Autodesk Fusion 360 part; units mm, degrees
(part 2 of 2)
sketch "side_face" plane through (8.1771, 0, 4.1664) normal (0.891007, 0, 0.45399) x (0, 1, 0) in component "sides"
  line L0 (-20, -43.5513) -> (-23, -43.5513)
  line L1 (-23, -43.5513) -> (-23, -35.5513)
  line L2 (-23, -35.5513) -> (-20, -35.5513)
  line L3 (-20, -35.5513) -> (-20, -43.5513)
  line L4 (20, -35.5513) -> (23, -35.5513)
  line L5 (23, -35.5513) -> (23, -43.5513)
  line L6 (23, -43.5513) -> (20, -43.5513)
  line L7 (20, -43.5513) -> (20, -35.5513)
  line L8 (22.4714, -88.3181) -> (61.9525, -140.4776)
  line L9 (61.9525, -140.4776) -> (67.9525, -140.4776)
  line L10 (67.9525, -140.4776) -> (67.9525, -143.8445)
  line L11 (67.9525, -143.8445) -> (73.9525, -143.8445)
  line L12 (73.9525, -143.8445) -> (73.9525, -140.4776)
  line L13 (73.9525, -140.4776) -> (23, -28.2449)
  line L14 (23, -28.2449) -> (-23, -28.2449)
  line L15 (-23, -28.2449) -> (-73.9525, -140.4776)
  line L16 (-73.9525, -140.4776) -> (-73.9525, -143.8445)
  line L17 (-73.9525, -143.8445) -> (-67.9525, -143.8445)
  line L18 (-67.9525, -143.8445) -> (-67.9525, -140.4776)
  line L19 (-67.9525, -140.4776) -> (-61.9525, -140.4776)
  line L20 (-61.9525, -140.4776) -> (-22.4714, -88.3181)
  ellipse E0 centre (-14.8502, -95.5845) end of major axis (-14.8502, -84.3612) minor radius 10 (-14.8502, -84.3612) -> (-22.4714, -88.3181) ccw
  line L21 (-14.8502, -84.3612) -> (14.8502, -84.3612)
  ellipse E1 centre (14.8502, -95.5845) end of major axis (14.8502, -84.3612) minor radius 10 (22.4714, -88.3181) -> (14.8502, -84.3612) ccw
sketch "base" plane through (0, 0, -121) normal (0, 0, 1) x (-1, 0, 0) in component "Base"
  line L0 (-62.5856, 70.2795) -> (-69.2795, 70.2795)
  line L1 (-69.2795, 70.2795) -> (-69.2795, 67.9525)
  line L2 (-69.2795, 67.9525) -> (-73.4811, 67.9525)
  line L3 (-73.4811, 67.9525) -> (-73.4811, 73.9525)
  line L4 (-73.4811, 73.9525) -> (-68.5856, 73.9525)
  line L5 (-68.5856, 73.9525) -> (-68.5856, 75.4811)
  line L6 (-68.5856, 75.4811) -> (-62.5856, 75.4811)
  line L7 (-62.5856, 75.4811) -> (-62.5856, 70.2795)
  line L8 (62.5856, 70.2795) -> (62.5856, 75.4811)
  line L9 (62.5856, 75.4811) -> (68.5856, 75.4811)
  line L10 (68.5856, 75.4811) -> (68.5856, 73.9525)
  line L11 (68.5856, 73.9525) -> (73.4811, 73.9525)
  line L12 (73.4811, 73.9525) -> (73.4811, 67.9525)
  line L13 (73.4811, 67.9525) -> (69.2795, 67.9525)
  line L14 (69.2795, 67.9525) -> (69.2795, 70.2795)
  line L15 (69.2795, 70.2795) -> (62.5856, 70.2795)
  line L16 (-62.5856, -70.2795) -> (-62.5856, -75.4811)
  line L17 (-62.5856, -75.4811) -> (-68.5856, -75.4811)
  line L18 (-68.5856, -75.4811) -> (-68.5856, -73.9525)
  line L19 (-68.5856, -73.9525) -> (-73.4811, -73.9525)
  line L20 (-73.4811, -73.9525) -> (-73.4811, -67.9525)
  line L21 (-73.4811, -67.9525) -> (-69.2795, -67.9525)
  line L22 (-69.2795, -67.9525) -> (-69.2795, -70.2795)
  line L23 (-69.2795, -70.2795) -> (-62.5856, -70.2795)
  line L24 (69.2795, -67.9525) -> (73.4811, -67.9525)
  line L25 (73.4811, -67.9525) -> (73.4811, -73.9525)
  line L26 (73.4811, -73.9525) -> (68.5856, -73.9525)
  line L27 (68.5856, -73.9525) -> (68.5856, -75.4811)
  line L28 (68.5856, -75.4811) -> (62.5856, -75.4811)
  line L29 (62.5856, -75.4811) -> (62.5856, -70.2795)
  line L30 (62.5856, -70.2795) -> (69.2795, -70.2795)
  line L31 (69.2795, -70.2795) -> (69.2795, -67.9525)
  circle A0 centre (0, 0) radius 85
  circle A1 centre (0, 0) radius 110
component "stepper" placed x (1, 0, 0) y (0, 1, 0) z (0, 0, 1) at (0, 0, 0)
component "front plate" placed x (1, 0, 0) y (0, 1, 0) z (0, 0, 1) at (0, 0, 0)
component "side plate" placed x (1, 0, 0) y (0, 1, 0) z (0, 0, 1) at (0, 0, 0)
component "front face" placed x (1, 0, 0) y (0, 1, 0) z (0, 0, 1) at (0, 0, 0)
component "sides" placed x (1, 0, 0) y (0, 1, 0) z (0, 0, 1) at (0, 0, 0)
component "Base" placed x (1, 0, 0) y (0, 1, 0) z (0, 0, 1) at (0, 0, 0)
hidden bodies 7 12 13
equation "d8 = d7"
equation "d9 = d7"
equation "d10 = d7"
equation "d74 = d25"
equation "d75 = d32"
equation "d97 = ( 23 / 2 ) * 1 mm"
equation "d98 = d97"
named bodies: "front face", "back face", "left_face", "right_face"
